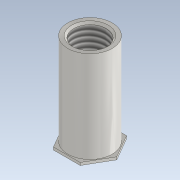
# Autodesk Inventor part: Вытяжная заклепка_Р-Ш-М5-Ум
Saved by Autodesk Inventor 2021.2 (Build 252289000, 289)
## iProperties
Created: 2009-05-22
Part Number: Вытяжная заклепка_Р-Ш-М5-Ум
Document SubType Name: Modeling
Designer: svb
Density: 7.85 g/cm^3
Material: Сталь низкоуглеродистая
Mass: 1.90299 g
Surface Area: 5.80512 cm^2
Volume: 0.242419 cm^3
Appearance: Сталь
Author: svb
Autodesk Inventor part; units mm, degrees
ref_plane "YZ Plane" through (0, 0, 0) normal (1, 0, 0) x (0, 1, 0)
ref_plane "XZ Plane" through (0, 0, 0) normal (0, 1, 0) x (-1, 0, 0)
ref_plane "XY Plane" through (0, 0, 0) normal (0, 0, 1) x (1, 0, 0)
sketch "Sketch1" plane through (0, 0, 0) normal (0, 0, 1) x (1, 0, 0)
  line L0 (2.0496, 3.55) -> (4.0992, 0)
  line L1 (4.0992, 0) -> (2.0496, -3.55)
  line L2 (2.0496, -3.55) -> (-2.0496, -3.55)
  line L3 (-2.0496, -3.55) -> (-4.0992, 0)
  line L4 (-4.0992, 0) -> (-2.0496, 3.55)
  line L5 (-2.0496, 3.55) -> (2.0496, 3.55)
  point P0 (0, 0)
  dimension "d0" = 7.1
  constraints: 12 end point, 13 other
  measures "d0" distance between parallel lines of L2 L5
extrude "Extrusion1" add sketch "Sketch1" along normal blind 0.4
sketch "Sketch2" plane through (0, 0, 0.4) normal (0, 0, 1) x (1, 0, 0)
  circle A0 centre (0, 0) radius 3.4
  dimension "d3" = 6.8
  constraints: 1 centre point
  measures "d3" diameter of A0
extrude "Extrusion2" add sketch "Sketch2" along normal blind 14
sketch "Sketch3" plane through (0, 0, 14.4) normal (0, 0, 1) x (1, 0, 0)
  circle A0 centre (0, 0) radius 3.4 projected
  circle A1 centre (0, 0) radius 2.5
  dimension "d6" = 5
  constraints: 1 centre point, 1 coincident
  measures "d6" diameter of A1
extrude "Extrusion3" cut sketch "Sketch3" against normal blind 15 contours A1
chamfer "Chamfer1" distance 0.3 angle 45 1 edges at (-2.5, 0, 14.4)
thread "Thread1" size "M5x0.8" class "6H" standard "ANSI Metric M Profile" full length
